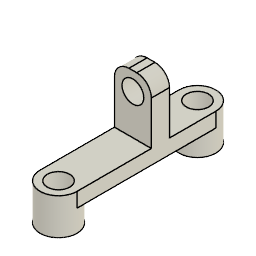
DriverSupport_v4 (Autodesk Fusion 360 design; units mm, degrees)
Autodesk Fusion 360 part; units mm, degrees
sketch "Sketch1" plane through (0, 0, 0) normal (0, 0, 1) x (1, 0, 0)
  line L0 (0, 11.075) -> (0, -11.075) construction
  line L1 (0, 8) -> (0, -8) construction
  circle A0 centre (0, 9.5375) radius 1.5375
  circle A1 centre (0, -9.5375) radius 1.5375
  circle A2 centre (0, 9.5375) radius 2.5375
  circle A3 centre (0, -9.5375) radius 2.5375
  line L2 (2.5375, 9.5375) -> (2.5375, -9.5375)
  line L3 (-2.5375, 9.5375) -> (-2.5375, -9.5375)
  dimension "d1" = 22.15
  dimension "d2" = 16
  dimension "d3" = 1
  dimension "d4" = 1
  constraint midpoint L0 origin
  constraint vertical L0
  constraint midpoint L1 origin
  constraint parallel L0 L1
  constraint coincident L1.start A0
  constraint coincident L0.start A0
  constraint coincident L1.end A1
  constraint coincident L0.end A1
  constraint concentric A0 A2
  constraint concentric A1 A3
  constraint coincident A2 L2.start
  constraint tangent A2 L2
  constraint parallel L0 L2
  constraint coincident A3 L2.end
  constraint tangent A3 L2
  constraint coincident A2 L3.start
  constraint coincident A3 L3.end
  constraint tangent A3 L3
  constraint vertical L3
  measures "d1" distance of L0.start L0.end
  measures "d2" distance of L1.start L1.end
  measures "d3" distance of A1 A3
  measures "d4" distance of A0 A2
extrude "Extrude1" add sketch "Sketch1" along normal blind 2
extrude "Extrude2" add sketch "Sketch1" against normal blind 3 contours A2 | A3
sketch "Sketch2" plane through (0, 0, 2) normal (0, 0, 1) x (-1, 0, 0)
  circle A0 centre (0, 9.5375) radius 1.5375
  circle A1 centre (0, -9.5375) radius 1.5375
  arc A2 (-2.5375, -9.5375) -> (2.5375, -9.5375) centre (0, -9.5375) ccw
  line L0 (2.5375, -9.5375) -> (2.5375, 9.5375)
  arc A3 (2.5375, 9.5375) -> (-2.5375, 9.5375) centre (0, 9.5375) ccw
  line L1 (-2.5375, 9.5375) -> (-2.5375, -9.5375)
  line L2 (2.5375, -3.1688) -> (-2.5375, -3.1688)
  line L3 (2.5375, -0.6688) -> (-2.5375, -0.6688)
  dimension "d9" = 2.5
  constraint coincident L0 L2.start
  constraint coincident L1 L2.end
  constraint perpendicular L1 L2
  constraint coincident L0 L3.start
  constraint coincident L1 L3.end
  constraint perpendicular L1 L3
  measures "d9" distance of L2 L3
extrude "Extrude3" add sketch "Sketch2" along normal blind 8 contours L0 L1 L2 L3
fillet "Fillet1" radius 2 2 edges at (2.5375, 1.9188, 10) (-2.5375, 1.9188, 10)
sketch "Sketch3" plane through (0, 3.1688, 0) normal (0, 1, 0) x (-1, 0, 0)
  arc A0 (2.5375, 8) -> (0.5375, 10) centre (0.5375, 8) ccw
  line L0 (0.5375, 10) -> (-0.5375, 10)
  arc A1 (-0.5375, 10) -> (-2.5375, 8) centre (-0.5375, 8) ccw
  line L1 (-2.5375, 8) -> (-2.5375, 2)
  line L2 (-2.5375, 2) -> (2.5375, 2)
  line L3 (2.5375, 2) -> (2.5375, 8)
  circle A2 centre (0, 7.5) radius 1.5
  line L4 (0, 10) -> (0, 7.5)
  dimension "d14" = 3
  dimension "d17" = 2.5
  constraint midpoint L0 L4.start
  constraint coincident A2.centre L4.end
  constraint perpendicular L0 L4
  measures "d14" diameter of A2
  measures "d17" distance of L4.start A2.centre
extrude "Extrude4" cut sketch "Sketch3" against normal blind 8 contours A2
